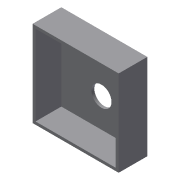
# Autodesk Inventor part: aanstuurkast
Saved by Autodesk Inventor 2019 (Build 230136000, 136)
## iProperties
Created: 2020-02-29
Part Number: aanstuurkast
Material: Generic
Document SubType Name: Modeling
Designer: stef_
Density: 1 g/cm^3
Appearance: Default
Author: stef_
Autodesk Inventor part; units mm, degrees
ref_plane "YZ Plane" through (0, 0, 0) normal (1, 0, 0) x (0, 1, 0)
ref_plane "XZ Plane" through (0, 0, 0) normal (0, 1, 0) x (-1, 0, 0)
ref_plane "XY Plane" through (0, 0, 0) normal (0, 0, 1) x (1, 0, 0)
sketch "Sketch1" plane through (0, 0, 0) normal (0, 0, 1) x (1, 0, 0)
  line L0 (-150, 74.8538) -> (150, 74.8538)
  line L1 (150, 74.8538) -> (150, -225.1462)
  line L2 (150, -225.1462) -> (-150, -225.1462)
  line L3 (-150, -225.1462) -> (-150, 74.8538)
  point P0 (0, 0)
  dimension "d0" = 300
  dimension "d1" = 300
  dimension "d2" = 150
  constraints: 8 end point, 2 parallel, 1 horizontal, 1 perpendicular
  measures "d0" distance of L1.end L2.end
  measures "d1" distance of L0.end L1.end
  measures "d2" distance from line of point (0, 0) L1
extrude "Extrusion1" add sketch "Sketch1" along normal blind 100
shell "Shell1" thickness 10 removed faces 1 at (-50, -25.1462, 100)
sketch "Sketch2" plane through (-140, 64.8538, 10) normal (0, 0, 1) x (1, 0, 0)
  circle A0 centre (140, -178.7412) radius 35 projected
  circle A1 centre (140, -178.7412) radius 35 projected
  circle A2 centre (140, -178.7412) radius 35
  point P0 (140, -64.8538)
  constraints: 1 centre point, 1 coincident, 1 concentric
extrude "Extrusion2" cut sketch "Sketch2" against normal up to next
sketch "Sketch3" plane through (0, 0, 100) normal (0, 0, 1) x (1, 0, 0)
  line L0 (-140, 64.8538) -> (140, 64.8538) projected
  line L1 (-150, 74.8538) -> (-150, -225.1462) projected
  line L2 (150, -225.1462) -> (150, 74.8538) projected
  line L3 (140, -215.1462) -> (-140, -215.1462) projected
  point P0 (0, 0)
  point P1 (-144, 68.8538)
  point P2 (144, 68.8538)
  point P3 (144, -219.1462)
  point P4 (-144, -219.1462)
  dimension "d8" = 4
  dimension "d9" = 6
  dimension "d10" = 6
  dimension "d11" = 6
  dimension "d12" = 6
  dimension "d13" = 4
  dimension "d14" = 4
  dimension "d15" = 4
  measures "d8" distance from line of L0 point (-144, 68.854)
  measures "d9" distance from line of L1 point (-144, 68.854)
  measures "d10" distance from line of L2 point (144, 68.854)
  measures "d11" distance from line of L2 point (144, -219.146)
  measures "d12" distance from line of L1 point (-144, -219.146)
  measures "d13" distance from line of L3 point (-144, -219.146)
  measures "d14" distance from line of L3 point (144, -219.146)
  measures "d15" distance from line of L0 point (144, 68.854)
hole "Hole1" at (-144, 68.8538, 100) at (144, 68.8538, 100) at (144, -219.1462, 100) at (-144, -219.1462, 100) direction (0, 0, -1) diameter 6.647 depth 22.2 tip angle 118 thread size "M8x1.25" class "6H" standard "ISO Metric profile"
body "Solid1"
